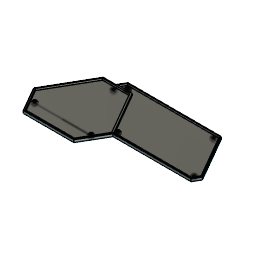
connecting-base (Autodesk Fusion 360 design; units mm, degrees)
part number: 2026-08-12-14-10-41-623
Autodesk Fusion 360 part; units mm, degrees
sketch "Sketch1" plane through (0, 0, 0) normal (0, 0, 1) x (1, 0, 0)
  line L0 (132.9156, -2.6788) -> (90.8719, 70.1431)
  line L1 (-68.2902, 57.6361) -> (-89, 57.6361)
  line L2 (-130.8761, -14.8954) -> (-107.7319, -54.9824)
  line L3 (-1.4217, -14.5431) -> (126, -14.5431)
  line L4 (126, -14.5431) -> (132.9156, -2.6788)
  line L5 (-61, 70.1431) -> (-68.2902, 57.6361)
  line L6 (-89, 57.6361) -> (-130.8761, -14.8954)
  line L7 (-106, -54.9824) -> (-24.9935, -54.9824)
  line L8 (-24.9935, -54.9824) -> (-1.4217, -14.5431)
  line L9 (90.8719, 70.1431) -> (-61, 70.1431)
  line L10 (-107.7319, -54.9824) -> (-106, -54.9824)
  point P0 (-65.7873, -4.2127)
  point P1 (-65.7873, -4.2127)
  point P2 (-65.7873, -4.2127)
  dimension "d4" = 94.1192
  dimension "d5" = 81.0065
  dimension "d6" = 14.5431
  dimension "d7" = 1.4217
  dimension "d8" = 125.1255
  dimension "d9" = 263.7917
  dimension "d10" = 120
  dimension "d11" = 120
  dimension "d12" = 120.238
  dimension "d13" = 234.5587
  dimension "d14" = 204.2045
  dimension "d15" = 151.8719
  dimension "d16" = 20.7098
  dimension "d17" = 46.8077
  dimension "d18" = 10.3305
  dimension "d19" = 64.3656
  constraint parallel L4 L8
  constraint parallel L4 L5
  constraint parallel L7 L10
  constraint coincident P2 P1
  constraint parallel L0 L2
  constraint parallel L1 L10
  constraint parallel L9 L10
  constraint parallel L3 L10
  constraint horizontal L10
  measures "d4" distance of L5 L8
  measures "d5" horizontal distance of L7.start L7.end
  measures "d6" distance of origin L3
  measures "d7" horizontal distance of origin L3.start
  measures "d8" distance of L7 L9
  measures "d9" horizontal distance of L0.start L2.start
  measures "d10" angle of L1 L6
  measures "d11" angle of L2 L10
  measures "d12" angle of L3 L4
  measures "d13" distance of L0 L2
  measures "d14" distance of L4 L5
  measures "d15" horizontal distance of L0.end L5.start
  measures "d16" horizontal distance of L1.start L1.end
  measures "d17" distance of L7.end L3.start
  measures "d18" distance of P2 L3
  measures "d19" horizontal distance of P2 L3.start
extrude "Extrude1" add sketch "Sketch1" along normal blind 2
sketch "Sketch2" plane through (0, 0, 2) normal (0, 0, 1) x (-1, 0, 0)
  line L0 (107.7319, 54.9824) -> (24.9935, 54.9824)
  line L1 (24.9935, 54.9824) -> (1.4217, 14.5431)
  line L2 (1.4217, 14.5431) -> (-126, 14.5431)
  line L3 (-126, 14.5431) -> (-132.9156, 2.6788)
  line L4 (-132.9156, 2.6788) -> (-90.8719, -70.1431)
  line L5 (-90.8719, -70.1431) -> (61, -70.1431)
  line L6 (61, -70.1431) -> (68.2902, -57.6361)
  line L7 (68.2902, -57.6361) -> (89, -57.6361)
  line L8 (89, -57.6361) -> (130.8761, 14.8954)
  line L9 (130.8761, 14.8954) -> (107.7319, 54.9824)
  line L10 (60.0858, -67.913) -> (-90.0874, -67.913)
  line L11 (-130.8139, 2.9274) -> (-125.2213, 12.6142)
  line L12 (25.7881, 52.8324) -> (3.6818, 14.5431)
  line L13 (-126, 14.5431) -> (-132.9156, 2.6788)
  line L14 (-125.3079, 12.7642) -> (1.418, 12.7642)
  line L15 (-90.8719, -70.1431) -> (61, -70.1431)
  line L16 (3.6818, 14.5431) -> (43.681, -54.7376)
  line L17 (1.4217, 14.5431) -> (-126, 14.5431)
  line L18 (25.7015, 52.9824) -> (3.5086, 14.5431)
  line L19 (3.5086, 14.5431) -> (43.5944, -54.8876)
  line L20 (1.3314, 12.6142) -> (41.949, -57.7376)
  line L21 (59.9992, -67.763) -> (-90.0008, -67.763)
  line L22 (-130.9871, 2.9274) -> (-125.3079, 12.7642)
  line L23 (-125.2213, 12.6142) -> (1.3314, 12.6142)
  line L24 (-90.0008, -67.763) -> (-130.8139, 2.9274)
  line L25 (87.8937, -54.7376) -> (43.681, -54.7376)
  line L26 (65.7873, 4.2127) -> (65.7873, -54.7376)
  line L27 (-90.0874, -67.913) -> (-130.9871, 2.9274)
  line L28 (106, 54.9824) -> (24.9935, 54.9824)
  line L29 (61, -70.1431) -> (68.2902, -57.6361)
  line L30 (68.2902, -57.6361) -> (89, -57.6361)
  line L31 (-132.9156, 2.6788) -> (-90.8719, -70.1431)
  line L32 (87.9803, -54.8876) -> (43.5944, -54.8876)
  line L33 (41.949, -57.7376) -> (65.7873, -57.7376)
  circle A0 centre (65.7873, 4.2127) radius 44.2127
  line L34 (25.7015, 52.9824) -> (105.8732, 52.9824)
  line L35 (42.0356, -57.5876) -> (66.0471, -57.5876)
  line L36 (65.7873, 4.2127) -> (14.7349, 33.6878)
  line L37 (107.7319, 54.9824) -> (106, 54.9824)
  line L38 (65.7873, 4.2127) -> (116.8397, 33.6878)
  line L39 (89, -57.6361) -> (130.8761, 14.8954)
  line L40 (130.8761, 14.8954) -> (107.7319, 54.9824)
  line L41 (128.0661, 14.5431) -> (105.8732, 52.9824)
  line L42 (66.0471, -57.5876) -> (60.0858, -67.913)
  line L43 (87.9803, -54.8876) -> (128.0661, 14.5431)
  line L44 (65.7873, -57.7376) -> (59.9992, -67.763)
  line L45 (127.8929, 14.5431) -> (105.7866, 52.8324)
  line L46 (87.8937, -54.7376) -> (127.8929, 14.5431)
  line L47 (65.7873, 4.2127) -> (65.7873, -84.2127) construction
  line L48 (25.7881, 52.8324) -> (105.7866, 52.8324)
  line L49 (65.7873, 4.2127) -> (65.7873, -84.2127) construction
  line L50 (1.418, 12.7642) -> (42.0356, -57.5876)
  line L51 (24.9935, 54.9824) -> (1.4217, 14.5431)
  point P0 (65.7873, 4.2127)
  point P1 (65.7873, 4.2127)
  point P2 (65.7873, 4.2127)
  dimension "d22" = -0.15
  dimension "d23" = 0.15
  dimension "d24" = 120
  dimension "d25" = 120
  dimension "d26" = 88.4253
  dimension "d27" = 62.1056
  dimension "d28" = 39.9992
  dimension "d29" = 22.1063
  dimension "d30" = 39.9992
  dimension "d31" = 29.4751
  dimension "d32" = 3
  dimension "d33" = 3
  dimension "d34" = 150
  dimension "d35" = 126.5527
  dimension "d36" = 196.6013
  dimension "d37" = 8.4015
  dimension "d38" = 12.6142
  dimension "d40" = 2
  dimension "d41" = 0.238
  dimension "d43" = 0.1015
  dimension "d44" = 20.052
  dimension "d45" = 1.9444
  dimension "d46" = 2.2813
  dimension "d47" = 9.9353
  dimension "d48" = 82.7572
  dimension "d49" = 94.1192
  dimension "d51" = 81.0065
  constraint coincident P2 P1
  constraint coincident L26.end L47
  constraint midpoint L36.end L12
  constraint perpendicular L12 L36
  constraint midpoint L38.end L45
  constraint perpendicular L38 L45
  constraint midpoint L26.end L25
  constraint perpendicular L25 L49
  constraint parallel L12 L46
  constraint coincident L47.end L49.end
  constraint parallel L25 L48
  constraint collinear L26 L49
  constraint parallel L16 L20
  constraint coincident L33.end L47
  constraint perpendicular L33 L47
  constraint perpendicular L21 L47
  constraint parallel L20 L24
  constraint parallel L21 L23
  constraint parallel L11 L12
  constraint parallel L44 L46
  constraint parallel L28 L34
  constraint parallel L17 L23
  constraint parallel L13 L51
  constraint parallel L27 L31
  constraint parallel L10 L15
  constraint parallel L13 L29
  constraint perpendicular L30 L47
  constraint parallel L39 L43
  constraint parallel L40 L45
  constraint parallel L28 L37
  constraint coincident L3.end L4.start
  constraint coincident L2.end L3.start
  constraint coincident L1.end L2.start
  measures "d24" angle of L38 L47
  measures "d25" angle of L36 L49
  measures "d26" diameter of A0
  measures "d27" distance of L12.end L26
  measures "d28" distance of L12.start L26
  measures "d29" distance of L16.end L26
  measures "d30" distance of L45.end L26
  measures "d31" distance of L47.end L25
  measures "d32" distance of L25 L33
  measures "d33" distance of L16 L20
  measures "d34" distance of L21.start L21.end
  measures "d35" distance of L11.end L20.start
  measures "d36" distance of L11.start L47
  measures "d37" distance of P2 L23
  measures "d38" distance of origin L23
  measures "d40" distance of L28 L34
  measures "d41" angle of L12 L51
  measures "d43" distance of L30 L33
  measures "d44" distance of L39 L44
  measures "d45" distance of L24 L31
  measures "d46" distance of L8.end L23
  measures "d47" distance of L3.end L23
  measures "d48" distance of L15 L23
  measures "d49" distance of L29 L51
  measures "d51" horizontal distance of L0.end L28.start
extrude "Extrude2" add sketch "Sketch2" along normal blind 3 contours L0 L1 L2 L3 L4 L5 L6 L7 L8 L9 L13 L15 L17 L28 L29 L30 L31 L37 L39 L40 L51
chamfer "Chamfer1" distance 0.8 angle 45 10 edges at (-109.9381, 21.3703, 5) (-78.6451, 57.6361, 5) (-64.6451, 63.8896, 5) (14.936, 70.1431, 5) (111.8938, 33.7321, 5) (129.4578, -8.611, 5) (62.2891, -14.5431, 5) (-13.2076, -34.7628, 5) (-119.304, -34.9389, 5) (-66.3627, -54.9824, 5)
sketch "Sketch3" plane through (0, 0, 0) normal (0, 0, -1) x (1, 0, 0)
  line L0 (-24.9935, 54.9824) -> (-107.7319, 54.9824)
  line L1 (-107.7319, 54.9824) -> (-130.8761, 14.8954)
  line L2 (-130.8761, 14.8954) -> (-89, -57.6361)
  line L3 (-89, -57.6361) -> (-68.2902, -57.6361)
  line L4 (-68.2902, -57.6361) -> (-61, -70.1431)
  line L5 (-61, -70.1431) -> (90.8719, -70.1431)
  line L6 (90.8719, -70.1431) -> (132.9156, 2.6788)
  line L7 (132.9156, 2.6788) -> (126, 14.5431)
  line L8 (126, 14.5431) -> (-1.4217, 14.5431)
  line L9 (-1.4217, 14.5431) -> (-24.9935, 54.9824)
  circle A0 centre (-113, 31) radius 1.7
  circle A1 centre (-20.4501, 31) radius 1.7
  line L10 (-113, 31) -> (-20.4501, 31)
  line L11 (-20.4501, 31) -> (-66.725, 31)
  circle A2 centre (-66, -51) radius 1.7
  circle A3 centre (122.1654, 5.5748) radius 1.7
  circle A4 centre (-2.8346, 5.5748) radius 1.7
  circle A5 centre (-55.8346, -64.4252) radius 1.7
  circle A6 centre (84.1654, -64.4252) radius 1.7
  point P0 (-2.8346, 5.5748)
  point P1 (-55.8346, -64.4252)
  dimension "d55" = 3.4
  dimension "d56" = 3.4
  dimension "d57" = 3.4
  dimension "d58" = 3.4
  dimension "d59" = 3.4
  dimension "d60" = 3.4
  dimension "d61" = 3.4
  dimension "d62" = 16.1046
  dimension "d63" = 253.0415
  dimension "d64" = 215.0415
  dimension "d65" = 128.0415
  dimension "d66" = 75.0415
  dimension "d67" = 64.8761
  dimension "d68" = 110.426
  dimension "d69" = 92.5499
  dimension "d70" = 79.3207
  dimension "d71" = 65.8954
  dimension "d72" = 9.3207
  constraint coincident A0.centre L10.start
  constraint coincident A1.centre L10.end
  constraint horizontal L10
  constraint midpoint L10 L11.end
  constraint coincident P0 A4.centre
  constraint coincident P1 A5.centre
  constraint horizontal P1 A6.centre
  constraint horizontal A3.centre P0
  measures "d55" diameter of A0
  measures "d56" diameter of A1
  measures "d57" diameter of A2
  measures "d58" diameter of A3
  measures "d59" diameter of A4
  measures "d60" diameter of A5
  measures "d61" diameter of A6
  measures "d62" distance of L1.end L10
  measures "d63" horizontal distance of L1.end A3.centre
  measures "d64" horizontal distance of L1.end A6.centre
  measures "d65" horizontal distance of L1.end P0
  measures "d66" horizontal distance of L1.end P1
  measures "d67" horizontal distance of L1.end A2.centre
  measures "d68" horizontal distance of L1.end A1.centre
  measures "d69" horizontal distance of A0.centre A1.centre
  measures "d70" vertical distance of L1.end P1
  measures "d71" vertical distance of L1.end A2.centre
  measures "d72" vertical distance of L1.end P0
extrude "Extrude4" cut sketch "Sketch3" against normal blind 1.5 contours A0 | A1 | A2 | A3 | A4 | A5 | A6
fillet "Fillet1" radius 0.5 7 edges at (-22.0351, -31.6147, 0) (-114.585, -31.6147, 0) (-67.585, 50.3853, 0) (-57.4195, 63.8105, 0) (-4.4195, -6.1895, 0) (120.5805, -6.1895, 0) (82.5805, 63.8105, 0)
